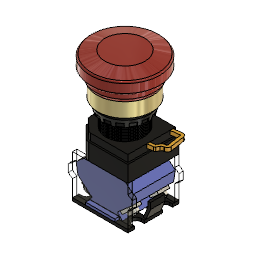
_EStop_LA38 _203 209B.204cfa63-6cc7-4e90-86a4-f45930ce202f (Autodesk Fusion 360 design; units mm, degrees)
Autodesk Fusion 360 part; units mm, degrees
sketch "Sketch1" plane through (0, 0, 0) normal (0, 0, 1) x (1, 0, 0)
  line L0 (16, 14.75) -> (-16, 14.75)
  line L1 (-16, -14.75) -> (16, -14.75)
  line L2 (16, 14.75) -> (-16, -14.75) construction
  line L3 (-16, 14.75) -> (16, -14.75) construction
  line L4 (16, -14.75) -> (16, -11)
  line L5 (16, -5.25) -> (14.375, -5.25)
  arc A0 (14.375, -5.25) -> (14.375, -11) centre (14.375, -8.125) ccw
  line L6 (16, -14.75) -> (16, -11)
  line L7 (16, -11) -> (14.375, -11)
  line L8 (14.25, 3) -> (8.25, 3)
  line L9 (8.25, 3) -> (8.25, -3)
  line L10 (8.25, -3) -> (14.25, -3)
  line L11 (14.25, -3) -> (14.25, 3)
  line L12 (0, -14.75) -> (0, 14.75) construction
  arc A1 (-14.375, -11) -> (-14.375, -5.25) centre (-14.375, -8.125) ccw
  line L13 (-16, -11) -> (-14.375, -11)
  line L14 (-16, -5.25) -> (-14.375, -5.25)
  line L15 (-8.25, -3) -> (-14.25, -3)
  line L16 (-14.25, -3) -> (-14.25, 3)
  line L17 (-14.25, 3) -> (-8.25, 3)
  line L18 (-8.25, 3) -> (-8.25, -3)
  line L19 (-16, 0) -> (16, 0) construction
  arc A2 (-14.375, 5.25) -> (-14.375, 11) centre (-14.375, 8.125) ccw
  line L20 (-16, 5.25) -> (-14.375, 5.25)
  line L21 (-16, 11) -> (-14.375, 11)
  line L22 (16, 11) -> (14.375, 11)
  arc A3 (14.375, 11) -> (14.375, 5.25) centre (14.375, 8.125) ccw
  line L23 (16, 5.25) -> (14.375, 5.25)
  line L24 (-16, 14.75) -> (-16, 11)
  line L25 (-16, 5.25) -> (-16, -5.25)
  line L26 (-16, -11) -> (-16, -14.75)
  line L27 (16, -14.75) -> (16, -11) construction
  line L28 (16, -5.25) -> (16, 5.25)
  line L29 (16, 11) -> (16, 14.75)
  line L30 (16, -5.25) -> (16, 5.25) construction
  line L31 (16, 11) -> (16, 14.75) construction
  dimension "d1" = 32
  dimension "d2" = 29.5
  dimension "d3" = 3.75
  dimension "d4" = 5.75
  dimension "d7" = 6
  dimension "d8" = 6
  constraint horizontal L0
  constraint perpendicular L0 L24
  constraint parallel L0 L1
  constraint parallel L6 L26
  constraint coincident L2 origin
  constraint coincident L3 origin
  constraint perpendicular L1 L4
  constraint perpendicular L5 L28
  constraint tangent L5 A0
  constraint tangent A0 L7
  constraint collinear L6 L28
  constraint horizontal L8
  constraint perpendicular L8 L9
  constraint parallel L8 L10
  constraint parallel L9 L11
  constraint midpoint L1 L12.start
  constraint midpoint L0 L12.end
  constraint symmetric L4.end L12 L13.start
  constraint symmetric L5.start L12 L14.start
  constraint symmetric L5.end L12 A1.end
  constraint symmetric A0 L12 A1
  constraint symmetric A0.end L12 A1.start
  constraint symmetric L8.start L12 L16.end
  constraint symmetric L8.end L12 L17.end
  constraint symmetric L9.end L12 L15.start
  constraint symmetric L10.end L12 L15.end
  constraint symmetric L4.end L19 L22.start
  constraint symmetric L5.start L19 L23.start
  constraint symmetric L5.end L19 A3.end
  constraint symmetric A0 L19 A3
  constraint symmetric A0.end L19 L22.end
  constraint symmetric A1.end L19 A2.start
  constraint symmetric A1.start L19 A2.end
  constraint symmetric A1 L19 A2
  constraint symmetric L13.start L19 L21.start
  constraint symmetric L14.start L19 L20.start
  constraint collinear L24 L25
  constraint collinear L25 L26
  constraint coincident L19.start L25
  constraint collinear L27 L30
  constraint collinear L28 L29
  constraint collinear L30 L31
  constraint coincident L19.end L30
  measures "d1" distance of L1.start L1.end
  measures "d2" distance of L0.end L1.start
  measures "d3" distance of L1.end L4.end
  measures "d4" distance of L4.end L5.start
  measures "d7" distance of L9.end L10.end
  measures "d8" distance of L8.end L9.end
extrude "Extrude1" add sketch "Sketch1" along normal blind 1.75 makes body 1
sketch "Sketch2" plane through (0, -14.75, 0) normal (0, -1, 0) x (1, 0, 0)
  line L0 (-16, 0) -> (16, 0)
  line L1 (16, 0) -> (16, 1.75)
  line L2 (16, 1.75) -> (-16, 1.75)
  line L3 (-16, 1.75) -> (-16, 0)
  line L4 (-16, 1.75) -> (16, 1.75)
  line L5 (16, 24.75) -> (-16, 24.75)
  line L6 (16, 1.75) -> (16, 11.25)
  line L7 (18.5, 13) -> (18.5, 17.5)
  line L8 (18.5, 13) -> (16, 11.25)
  line L9 (18.5, 17.5) -> (16, 19.25)
  line L10 (0, 1.75) -> (0, 24.75) construction
  line L11 (16, 1.75) -> (16, 11.25)
  line L12 (16, 19.25) -> (16, 24.75)
  line L13 (-18.5, 13) -> (-16, 11.25)
  line L14 (-18.5, 13) -> (-18.5, 17.5)
  line L15 (-18.5, 17.5) -> (-16, 19.25)
  line L16 (-16, 24.75) -> (-16, 19.25)
  line L17 (-16, 11.25) -> (-16, 1.75)
  dimension "d11" = 23
  dimension "d12" = 9.5
  dimension "d15" = 4.5
  constraint horizontal L4
  constraint vertical L11
  constraint horizontal L5
  constraint vertical L16
  constraint coincident L2.end L3.start
  constraint coincident L1.end L2.start
  constraint perpendicular L2 L6
  constraint midpoint L2 L10.start
  constraint midpoint L5 L10.end
  constraint perpendicular L5 L10
  constraint collinear L11 L12
  constraint symmetric L6.end L10 L13.end
  constraint symmetric L7.start L10 L13.start
  constraint symmetric L7.end L10 L14.end
  constraint symmetric L9.end L10 L15.end
  constraint collinear L16 L17
  measures "d11" distance of L2.end L5.end
  measures "d12" distance of L1.end L6.end
  measures "d15" distance of L7.start L7.end
extrude "Extrude1'" add sketch "Sketch2" against normal blind 2.5 separate body contours L2 L4 L5 L6 L7 L8 L9 L11 L12 L13 L14 L15 L16 L17 makes body 2 in component "Acryllic Panels"
ref_plane "WorkPlane1" through (0, 0, 0.875) normal (0, 1, 0) x (-1, 0, 0)
mirror "Mirror1" about plane through (0, 0, 0.875) normal (0, 1, 0) of bodies 2 makes body 3 in component "Acryllic Panels"
sketch "Sketch3" plane through (0, -12.25, 0) normal (0, -1, 0) x (1, 0, 0)
  line L0 (-18.5, 13) -> (-16, 11.25)
  line L1 (-16, 11.25) -> (-16, 1.75)
  line L2 (-16, 1.75) -> (16, 1.75)
  line L3 (16, 1.75) -> (16, 11.25)
  line L4 (16, 11.25) -> (18.5, 13)
  line L5 (18.5, 13) -> (18.5, 17.5)
  line L6 (18.5, 17.5) -> (16, 19.25)
  line L7 (16, 19.25) -> (16, 24.75)
  line L8 (16, 24.75) -> (-16, 24.75)
  line L9 (-16, 24.75) -> (-16, 19.25)
  line L10 (-16, 19.25) -> (-18.5, 17.5)
  line L11 (-18.5, 17.5) -> (-18.5, 13)
  line L12 (-16, 0) -> (16, 0)
  line L13 (16, 0) -> (16, 1.75)
  line L14 (16, 1.75) -> (-16, 1.75)
  line L15 (-16, 1.75) -> (-16, 0)
  line L16 (-10.125, 1.75) -> (10.125, 1.75)
  line L17 (0, 1.75) -> (0, 6.5)
  line L18 (-6, 6.5) -> (6, 6.5)
  line L19 (-10.125, 1.75) -> (-6, 6.5)
  line L20 (6, 6.5) -> (10.125, 1.75)
  line L21 (-8.5, 1.75) -> (8.5, 1.75)
  line L22 (-8.5, 1.75) -> (8.5, 1.75)
  line L23 (8.5, 1.75) -> (8.5, 3.25)
  line L24 (8.5, 3.25) -> (-8.5, 3.25)
  line L25 (-8.5, 3.25) -> (-8.5, 1.75)
  line L26 (-6, 6.5) -> (-6, 12) construction
  line L27 (-18.5, 14) -> (-15.5, 14) construction
  line L28 (-15.5, 12) -> (-7.3614, 4.9323)
  line L29 (-15.5, 12) -> (-16.5, 18.25)
  line L30 (-9, 24.75) -> (-16.5, 18.25)
  line L31 (15.5, 12) -> (7.3614, 4.9323)
  line L32 (15.5, 12) -> (16.5, 18.25)
  line L33 (9, 24.75) -> (16.5, 18.25)
  line L34 (-9, 24.75) -> (9, 24.75)
  line L35 (-16, 11.25) -> (-18.5, 13)
  line L36 (-18.5, 13) -> (-18.5, 17.5)
  line L37 (-18.5, 17.5) -> (-16, 19.25)
  line L38 (-16, 19.25) -> (-16, 24.75)
  line L39 (-16, 24.75) -> (16, 24.75)
  line L40 (16, 24.75) -> (16, 19.25)
  line L41 (16, 19.25) -> (18.5, 17.5)
  line L42 (18.5, 17.5) -> (18.5, 13)
  line L43 (18.5, 13) -> (16, 11.25)
  line L44 (16, 11.25) -> (16, 1.75)
  line L45 (16, 1.75) -> (-16, 1.75)
  line L46 (-16, 1.75) -> (-16, 11.25)
  point P0 (0, 1.75)
  point P1 (0, 1.75)
  dimension "d20" = 20.25
  dimension "d21" = 4.75
  dimension "d22" = 12
  dimension "d23" = 17
  dimension "d24" = 1.5
  dimension "d25" = 5.5
  dimension "d26" = 3
  constraint midpoint L16 P1
  constraint coincident L14 P1
  constraint parallel L2 L16
  constraint coincident P1 P0
  constraint perpendicular L2 L17
  constraint midpoint L17.end L18
  constraint perpendicular L17 L18
  constraint midpoint L21 P1
  constraint perpendicular L17 L21
  constraint horizontal L22
  constraint vertical L23
  constraint horizontal L24
  constraint vertical L25
  constraint perpendicular L18 L26
  constraint coincident L11 L27.start
  constraint perpendicular L11 L27
  constraint coincident L19 L28.end
  constraint perpendicular L19 L28
  constraint coincident L8 L30.start
  constraint symmetric L17 L28.start L31.start
  constraint symmetric L17 L28.end L31.end
  constraint symmetric L17 L29.end L32.end
  constraint symmetric L17 L30.start L33.start
  measures "d20" distance of L16.start L16.end
  measures "d21" distance of P1 L17.end
  measures "d22" distance of L18.start L18.end
  measures "d23" distance of L21.start L21.end
  measures "d24" distance of L21.start L24.end
  measures "d25" distance of L18.start L26.end
  measures "d26" distance of L27.start L27.end
extrude "Extrude2" cut sketch "Sketch3" along normal blind 2.5 contours L2 L14 L16 L17 L21 L22 L24 L25 L45 | L2 L14 L16 L17 L21 L22 L23 L24 L45 bodies 2 in component "Acryllic Panels"
extrude "Extrude1''" add sketch "Sketch3" along normal blind 2.5 separate body contours L2 L14 L16 L17 L21 L22 L24 L25 L45 | L2 L14 L16 L17 L21 L22 L23 L24 L45 makes body 4 in component "Inner Mechanism Block"
extrude "Extrude2'" add sketch "Sketch3" against normal blind 12.25 contours L2 L14 L16 L17 L18 L19 L24 L25 L45 | L2 L14 L16 L17 L21 L22 L24 L25 L45 | L8 L18 L19 L20 L28 L29 L30 L31 L32 L33 L34 L39 | L2 L14 L16 L17 L21 L22 L23 L24 L45 | L2 L14 L16 L17 L18 L20 L23 L24 L45 bodies 4 in component "Inner Mechanism Block"
mirror "Mirror1'" about plane through (0, 0, 0.875) normal (0, 1, 0) of bodies 4 merged in component "Inner Mechanism Block"
copy_body "Body->Comp1" bodies 1 removing the originals makes body 5 in component "Bottom Base"
sketch "Sketch4" plane through (0, 0, 0) normal (0, 1, 0) x (1, 0, 0)
  line L0 (-8.25, 0) -> (-8.25, -1.75)
  line L1 (-8.25, -1.75) -> (8.25, -1.75)
  line L2 (8.25, -1.75) -> (8.25, 0)
  line L3 (8.25, 0) -> (-8.25, 0)
  line L4 (16, -1.75) -> (16, 0)
  line L5 (16, 0) -> (14.25, 0)
  line L6 (14.25, 0) -> (14.25, -1.75)
  line L7 (14.25, -1.75) -> (16, -1.75)
  line L8 (-16, 0) -> (-16, -1.75)
  line L9 (-16, -1.75) -> (-14.25, -1.75)
  line L10 (-14.25, -1.75) -> (-14.25, 0)
  line L11 (-14.25, 0) -> (-16, 0)
  line L12 (-16, -1.75) -> (-16, -7.75)
  line L13 (-16, -7.75) -> (-18.5, -7.75)
  line L14 (-16, -1.75) -> (-18.5, -7.75)
  line L15 (-18.5, -7.75) -> (-18.5, -11.25)
  line L16 (-17, -8.05) -> (-17, -11.25)
  line L17 (-18.5, -11.25) -> (-17, -11.25)
  line L18 (-14.25, -1.75) -> (-17, -8.05)
  line L19 (0, -1.75) -> (0, -4) construction
  line L20 (14.25, -1.75) -> (17, -8.05)
  line L21 (16, -1.75) -> (18.5, -7.75)
  line L22 (17, -8.05) -> (17, -11.25)
  line L23 (18.5, -7.75) -> (18.5, -11.25)
  line L24 (18.5, -11.25) -> (17, -11.25)
  dimension "d37" = 6
  dimension "d38" = 2.5
  dimension "d39" = 3.5
  dimension "d40" = -1.5
  constraint coincident L8.end L9.start
  constraint perpendicular L9 L12
  constraint perpendicular L12 L13
  constraint perpendicular L13 L15
  constraint perpendicular L16 L17
  constraint coincident L9.end L10.start
  constraint midpoint L1 L19.start
  constraint perpendicular L1 L19
  constraint symmetric L13.end L19 L21.end
  constraint symmetric L8.end L19 L4.start
  constraint symmetric L15.end L19 L23.end
  constraint symmetric L16.start L19 L20.end
  constraint symmetric L16.end L19 L22.end
  constraint symmetric L9.end L19 L6.end
  measures "d37" distance of L8.end L12.end
  measures "d38" distance of L12.end L13.end
  measures "d39" distance of L13.end L15.end
extrude "Extrude1'''" add sketch "Sketch4" along normal mid plane 8.4 contours L7 L20 L21 L22 L23 L24 | L9 L12 L18 | L12 L13 L14 L18 | L13 L15 L16 L17 L18 bodies 5 in component "Bottom Base"
sketch "Sketch5" plane through (0, -14.75, 0) normal (0, -1, 0) x (1, 0, 0)
  line L0 (8.5, 3.25) -> (8.5, 1.75)
  line L1 (8.5, 1.75) -> (16, 1.75)
  line L2 (16, 1.75) -> (16, 11.25)
  line L3 (16, 11.25) -> (18.5, 13)
  line L4 (18.5, 13) -> (18.5, 17.5)
  line L5 (18.5, 17.5) -> (16, 19.25)
  line L6 (16, 19.25) -> (16, 24.75)
  line L7 (16, 24.75) -> (-16, 24.75)
  line L8 (-16, 24.75) -> (-16, 19.25)
  line L9 (-16, 19.25) -> (-18.5, 17.5)
  line L10 (-18.5, 17.5) -> (-18.5, 13)
  line L11 (-18.5, 13) -> (-16, 11.25)
  line L12 (-16, 11.25) -> (-16, 1.75)
  line L13 (-16, 1.75) -> (-8.5, 1.75)
  line L14 (-8.5, 1.75) -> (-8.5, 3.25)
  line L15 (-8.5, 3.25) -> (8.5, 3.25)
  line L16 (-16, 1.75) -> (16, 1.75)
  line L17 (-16, 0) -> (16, 0)
  line L18 (16, 0) -> (16, 1.75)
  line L19 (16, 1.75) -> (-16, 1.75)
  line L20 (-16, 1.75) -> (-16, 0)
extrude "Extrude3" cut sketch "Sketch5" against normal blind 29.5 contours L0 L14 L15 L16 L19 bodies 3 in component "Acryllic Panels"
ref_plane "WorkPlane2" through (14.2174, 0, 5.2573) normal (0.655687, 0, -0.755033) x (-0.755033, 0, -0.655687)
sketch "Sketch6" plane through (3.5097, 0, -4.0415) normal (0.655687, 0, -0.755033) x (-0.755033, 0, -0.655687)
  line L0 (-19.5713, -12.25) -> (-8.7922, -12.25)
  line L1 (-8.7922, -12.25) -> (-8.7922, 12.25)
  line L2 (-8.7922, 12.25) -> (-19.5713, 12.25)
  line L3 (-19.5713, 12.25) -> (-19.5713, -12.25)
  ellipse E0 centre (-10.8536, -8.125) end of major axis (-10.8536, -5.25) minor radius 2.1707 (-10.8536, -11) -> (-10.8536, -5.25) ccw
  line L4 (-10.8536, -8.125) -> (-8.7922, -8.125)
  line L5 (-8.7922, -8.125) -> (-13.0422, -8.125)
  circle A0 centre (-13.0422, -8.125) radius 2.75
  line L6 (-8.7922, 0) -> (-10.2486, 0) construction
  circle A1 centre (-13.0422, 8.125) radius 2.75
  dimension "d46" = 4.25
  dimension "d47" = 5.5
  constraint coincident E0.centre L4.start
  constraint coincident L1 L4.end
  constraint perpendicular L1 L4
  constraint perpendicular L1 L5
  constraint coincident L5.end A0.centre
  constraint midpoint L1 L6.start
  constraint perpendicular L1 L6
  constraint symmetric A0 L6 A1
  measures "d46" distance of L4.end L5.end
  measures "d47" diameter of A0
extrude "Extrude1''''" add sketch "Sketch6" against normal blind 4.25 separate body contours A0 | A1 makes body 6 at (10.3621, 7.8512, 3.7855) makes body 7 at (9.4254, -8.2621, 4.8484) in component "Screw Terminals"
ref_plane "WorkPlane3" through (11.7178, 8.125, 6.3977) normal (0.655687, 0, -0.755033) x (-0.755033, 0, -0.655687)
sketch "Sketch7" plane through (1.8705, 0, -2.1539) normal (0.655687, 0, -0.755033) x (-0.755033, 0, -0.655687)
  circle A0 centre (-13.0422, 8.125) radius 2.75
  circle A1 centre (-13.0422, -8.125) radius 2.75
  line L0 (-16.2922, -4.875) -> (-9.7922, -4.875)
  line L1 (-9.7922, -4.875) -> (-9.7922, -11.375)
  line L2 (-9.7922, -11.375) -> (-16.2922, -11.375)
  line L3 (-16.2922, -11.375) -> (-16.2922, -4.875)
  line L4 (-16.2922, -4.875) -> (-9.7922, -11.375) construction
  line L5 (-9.7922, -4.875) -> (-16.2922, -11.375) construction
  line L6 (-16.2922, 11.375) -> (-9.7922, 11.375)
  line L7 (-9.7922, 11.375) -> (-9.7922, 4.875)
  line L8 (-9.7922, 4.875) -> (-16.2922, 4.875)
  line L9 (-16.2922, 4.875) -> (-16.2922, 11.375)
  line L10 (-16.2922, 11.375) -> (-9.7922, 4.875) construction
  line L11 (-9.7922, 11.375) -> (-16.2922, 4.875) construction
  point P0 (-13.0422, -8.125)
  point P1 (-13.0422, 8.125)
  dimension "d51" = 6.5
  dimension "d52" = 6.5
  dimension "d53" = 6.5
  dimension "d54" = 6.5
  constraint horizontal L0
  constraint perpendicular L0 L1
  constraint parallel L0 L2
  constraint parallel L1 L3
  constraint coincident L4 P0
  constraint coincident L5 P0
  constraint coincident P0 A1.centre
  constraint horizontal L6
  constraint perpendicular L6 L7
  constraint parallel L6 L8
  constraint parallel L7 L9
  constraint coincident L10 P1
  constraint coincident L11 P1
  constraint coincident A0.centre P1
  measures "d51" distance of L1.end L2.end
  measures "d52" distance of L0.end L1.end
  measures "d53" distance of L7.end L8.end
  measures "d54" distance of L6.end L7.end
extrude "Extrude2''" cut sketch "Sketch7" against normal blind 1.75 contours A0 | A1 bodies 6 7 in component "Screw Terminals"
extrude "Extrude3'" add sketch "Sketch7" against normal blind 1.75 contours A0 | A1 | L0 L1 L2 L3 | L6 L7 L8 L9 bodies 6 7 in component "Screw Terminals"
sketch "Sketch8" plane through (3.5097, 0, -4.0415) normal (0.655687, 0, -0.755033) x (0, 1, 0)
  circle A0 centre (-8.125, 13.0422) radius 2.75
  circle A1 centre (8.125, 13.0422) radius 2.75
  line L0 (-8.75, 16) -> (-7.5565, 10.3516) construction
  line L1 (-5.404, 13.4408) -> (-10.846, 12.6435) construction
  line L2 (-8.125, 13.0422) -> (8.125, 13.0422)
  line L3 (0, 13.0422) -> (0, 14.5)
  line L4 (7.5, 10.0843) -> (7.5, 16)
  line L5 (8.75, 16) -> (8.75, 10.0843)
  line L6 (7.5, 16) -> (8.75, 16)
  line L7 (8.75, 10.0843) -> (7.5, 10.0843)
  line L8 (11.25, 12.5843) -> (5, 12.5843)
  line L9 (5, 13.5) -> (11.25, 13.5)
  line L10 (5, 12.5843) -> (5, 13.5)
  line L11 (-8.75, 15.7202) -> (-8.75, 13.5)
  line L12 (-8.75, 12.5843) -> (-8.75, 10.3641)
  line L13 (-5.4134, 13.5) -> (-7.5, 13.5)
  line L14 (-8.75, 13.5) -> (-10.8366, 13.5)
  line L15 (-7.5, 16) -> (-8.125, 13.0422) construction
  line L16 (-8.2217, 12.5843) -> (-8.6935, 10.3516) construction
  line L17 (-10.8366, 12.5843) -> (-8.75, 12.5843)
  line L18 (-7.5, 12.5843) -> (-5.4134, 12.5843)
  line L19 (-10.846, 13.4408) -> (-7.5, 12.9506) construction
  line L20 (-5.404, 12.6435) -> (-5, 12.5843) construction
  line L21 (-7.5, 10.3641) -> (-7.5, 12.5843)
  line L22 (-7.5, 12.9506) -> (-7.5, 15.7202)
  point P0 (-8.125, 13.0422)
  point P1 (-8.125, 13.0422)
  constraint parallel L11 L22
  constraint coincident P1 L15
  constraint coincident L0 P1
  constraint coincident P0 A0.centre
  constraint horizontal L13
  constraint parallel L13 L18
  constraint coincident L1 P1
  constraint coincident P1 L19
  constraint coincident P1 P0
  constraint coincident A1.centre L2.end
  constraint midpoint L2 L3.start
  constraint perpendicular L2 L3
  constraint symmetric L15.start L3 L4.end
  constraint symmetric L0.start L3 L5.start
  constraint symmetric L20.end L3 L8.end
  constraint coincident A0 L11.start
  constraint coincident A0 L22.end
  constraint coincident L13.end L22
  constraint collinear L15 L16
  constraint collinear L17 L18
  constraint coincident A0 L19.start
  constraint coincident A0 L14.end
  constraint coincident A0 L17.start
  constraint coincident A0 L1.end
  constraint coincident A0 L16.end
  constraint coincident A0 L0.end
  constraint coincident A0 L21.start
  constraint coincident A0 L12.end
  constraint coincident A0 L18.end
  constraint coincident A0 L1.start
  constraint coincident A0 L13.start
  constraint coincident A0 L20.start
  constraint collinear L19 L20
  constraint collinear L21 L22
extrude "Extrude4" cut sketch "Sketch8" against normal blind 0.75 contours A0 L2 L13 L22 | A0 L2 L11 L12 L14 L17 L18 L21 L22 | A1 L5 L8 L9 | A1 L4 L5 L9 | L4 L5 L8 L9 | A1 L4 L5 L8 | A1 L2 L4 L9 | A1 L2 L4 L8 bodies 6 7 in component "Screw Terminals"
chamfer "Chamfer1" distance 0.75 angle 45 8 edges at (14.779, -10.1289, 5.7449) (14.779, -6.1211, 5.7449) (11.935, -6.1211, 3.2752) (11.935, -10.1289, 3.2752) (14.779, 6.1211, 5.7449) (11.935, 6.1211, 3.2752) (11.935, 10.1289, 3.2752) (14.779, 10.1289, 5.7449) on bodies 6 7 in component "Screw Terminals"
ref_plane "WorkPlane4" through (0, 0, 0.875) normal (1, 0, 0) x (0, 1, 0)
mirror "Mirror1''" about plane through (0, 0, 0.875) normal (1, 0, 0) of bodies 6 7 makes body 8 at (-11.3883, 9.2083, 8.4293) makes body 9 at (-11.3883, -7.0417, 8.4293) in component "Screw Terminals"
sketch "Sketch9" plane through (0, 0, 24.75) normal (0, 0, 1) x (-1, 0, 0)
  line L0 (9, 12.25) -> (-9, 12.25)
  line L1 (-9, 12.25) -> (-9, -12.25)
  line L2 (-9, -12.25) -> (9, -12.25)
  line L3 (9, -12.25) -> (9, 12.25)
  line L4 (-16, -14.75) -> (16, -14.75)
  line L5 (16, -14.75) -> (16, -12.25)
  line L6 (16, -12.25) -> (-16, -12.25)
  line L7 (-16, -12.25) -> (-16, -14.75)
  line L8 (16, 14.75) -> (-16, 14.75)
  line L9 (-16, 14.75) -> (-16, 12.25)
  line L10 (-16, 12.25) -> (16, 12.25)
  line L11 (16, 12.25) -> (16, 14.75)
  line L12 (16, -12.25) -> (16, 12.25)
  line L13 (16, 7) -> (16, -7)
  line L14 (16, 0) -> (-9, 0) construction
  line L15 (-16, 12.25) -> (8, 12.25)
  line L16 (16, -7) -> (16, 7)
  line L17 (-16, 12.25) -> (8, 12.25)
  line L18 (-16, 12.25) -> (-16, -12.25)
  line L19 (-16, -14.75) -> (6.5827, -14.75)
  line L20 (-16, 14.75) -> (6.5827, 14.75)
  line L21 (9.018, 13.7638) -> (16, 7)
  line L22 (16, -7) -> (9.018, -13.7638)
  arc A0 (9.018, 13.7638) -> (6.5827, 14.75) centre (6.5827, 11.25) ccw
  arc A1 (6.5827, -14.75) -> (9.018, -13.7638) centre (6.5827, -11.25) ccw
  point P0 (16, 0)
  point P1 (8, -14.75)
  point P2 (8, 14.75)
  dimension "d65" = 14
  dimension "d66" = 24
  dimension "d67" = 24
  dimension "d68" = 3.5
  constraint coincident L6.end L7.start
  constraint coincident L5.end L6.start
  constraint coincident L10.end L11.start
  constraint midpoint L13 P0
  constraint coincident L12 P0
  constraint parallel L12 L13
  constraint coincident P0 L14.start
  constraint midpoint L1 L14.end
  constraint perpendicular L1 L14
  constraint symmetric L6.end L14 L9.end
  constraint symmetric L13.start L14 L13.end
  constraint symmetric L13.end L14 L13.start
  constraint coincident L9.end L10.start
  constraint coincident L4.start L7.end
  constraint perpendicular L7 L19
  constraint coincident L8.end L9.start
  constraint perpendicular L9 L20
  constraint coincident P2 L20
  constraint coincident P2 L21
  constraint tangent L20 A0
  constraint tangent L21 A0
  constraint coincident P1 L22
  constraint coincident P1 L19
  constraint tangent L22 A1
  constraint tangent L19 A1
  constraint equal A0 A1
  measures "d65" distance of L13.start L13.end
  measures "d66" distance of L4.start P1
  measures "d67" distance of L8.end P2
  measures "d68" radius of A0
extrude "Extrude1'''''" add sketch "Sketch9" along normal blind 9.5 separate body contours L0 L1 L2 L3 L6 L10 L15 L17 | L3 L6 L10 L12 L13 L16 L21 L22 | L0 L8 L9 L10 L15 L17 L20 L21 A0 | L2 L4 L6 L7 L19 L22 A1 | L1 L6 L10 L15 L17 L18 makes body 10 in component "Main Block"
sketch "Sketch10" plane through (0, 0, 34.25) normal (0, 0, 1) x (-1, 0, 0)
  line L0 (-16, 14.75) -> (-16, -14.75)
  line L1 (-16, -14.75) -> (6.5827, -14.75)
  arc A0 (6.5827, -14.75) -> (9.018, -13.7638) centre (6.5827, -11.25) ccw
  line L2 (9.018, -13.7638) -> (16, -7)
  line L3 (16, -7) -> (16, 7)
  line L4 (16, 7) -> (9.018, 13.7638)
  arc A1 (9.018, 13.7638) -> (6.5827, 14.75) centre (6.5827, 11.25) ccw
  line L5 (6.5827, 14.75) -> (-16, 14.75)
  line L6 (6.5827, 13.75) -> (-15, 13.75)
  line L7 (-15, 13.75) -> (-15, -13.75)
  line L8 (-15, -13.75) -> (6.5827, -13.75)
  arc A2 (6.5827, -13.75) -> (8.3222, -13.0456) centre (6.5827, -11.25) ccw
  line L9 (8.3222, -13.0456) -> (15, -6.5765)
  line L10 (15, -6.5765) -> (15, 6.5765)
  line L11 (15, 6.5765) -> (8.3222, 13.0456)
  arc A3 (8.3222, 13.0456) -> (6.5827, 13.75) centre (6.5827, 11.25) ccw
  dimension "d71" = -1
extrude "Extrude2'''" add sketch "Sketch10" along normal blind 4 contours L6 L7 L8 A2 L9 L10 L11 A3 bodies 10 in component "Main Block"
extrude "Extrude3''" cut 1 faces at (-2.4538, -12.25, 18.1441) along direction (0, 1, 0) blind 0.1 on bodies 4 bodies 4 in component "Inner Mechanism Block"
extrude "Extrude4'" cut 1 faces at (-2.4538, 12.25, 18.1441) along direction (0, -1, 0) blind 0.1 on bodies 4 bodies 4 in component "Inner Mechanism Block"
sketch "Sketch11" plane through (0, 0, 38.25) normal (0, 0, 1) x (-1, 0, 0)
  arc A0 (8.3222, 13.0456) -> (6.5827, 13.75) centre (6.5827, 11.25) ccw
  line L0 (6.5827, 13.75) -> (-15, 13.75)
  line L1 (-15, 13.75) -> (-15, -13.75)
  line L2 (-15, -13.75) -> (6.5827, -13.75)
  arc A1 (6.5827, -13.75) -> (8.3222, -13.0456) centre (6.5827, -11.25) ccw
  line L3 (8.3222, -13.0456) -> (15, -6.5765)
  line L4 (15, -6.5765) -> (15, 6.5765)
  line L5 (15, 6.5765) -> (8.3222, 13.0456)
  line L6 (15, 0) -> (1, 0)
  circle A2 centre (1, 0) radius 10.75
  dimension "d78" = 14
  dimension "d79" = 21.5
  constraint midpoint L4 L6.start
  constraint perpendicular L4 L6
  constraint coincident L6.end A2.centre
  measures "d78" distance of L6.start L6.end
  measures "d79" diameter of A2
extrude "Extrude1''''''" add sketch "Sketch11" along normal blind 8.5 separate body contours A2 makes body 11 in component "Button Threaded Base"
sketch "Sketch12" plane through (0, 0, 46.75) normal (0, 0, 1) x (-1, 0, 0)
  circle A0 centre (1, 0) radius 10.75
  circle A1 centre (1, 0) radius 13
  dimension "d82" = 26
  constraint concentric A0 A1
  measures "d82" diameter of A1
ref_plane "WorkPlane5" through (-1, 0, 51.25) normal (0, 0, 1) x (-1, 0, 0)
sketch "Sketch13" plane through (0, 0, 51.25) normal (0, 0, 1) x (1, 0, 0)
  circle A0 centre (-1, 0) radius 14.125
  dimension "d84" = 28.25
  measures "d84" diameter of A0
loft "Loft1" add profiles "Sketch12", "Sketch13" section 1 contours A0 | A1 section 2 bodies 11 in component "Button Threaded Base"
extrude "Extrude2''''" add 1 faces at (0.1003, -3.8885, 51.25) along direction (0, 0, 1) blind 2 on bodies 11 bodies 11 in component "Button Threaded Base"
sketch "Sketch14" plane through (0, 13.75, 0) normal (0, 1, 0) x (-1, 0, 0)
  line L0 (-15, 34.25) -> (6.5827, 34.25)
  line L1 (6.5827, 34.25) -> (6.5827, 38.25)
  line L2 (6.5827, 38.25) -> (-15, 38.25)
  line L3 (-15, 38.25) -> (-15, 34.25)
  line L4 (14, 46.75) -> (-12, 46.75)
  line L5 (-13.125, 51.25) -> (15.125, 51.25)
  line L6 (-12, 46.75) -> (14, 46.75)
  line L7 (1, 46.75) -> (1, 49.25)
  line L8 (2.75, 49.25) -> (-0.75, 49.25)
  line L9 (-0.75, 49.25) -> (-0.75, 46.75)
  line L10 (-0.75, 46.75) -> (2.75, 46.75)
  line L11 (2.75, 46.75) -> (2.75, 49.25)
  line L12 (2.75, 49.25) -> (-0.75, 46.75) construction
  line L13 (-0.75, 49.25) -> (2.75, 46.75) construction
  point P0 (1, 48)
  dimension "d87" = 2.5
  dimension "d88" = 3.5
  constraint coincident L4.end L6.start
  constraint coincident L4.start L6.end
  constraint midpoint L4 L7.start
  constraint perpendicular L6 L7
  constraint horizontal L8
  constraint perpendicular L8 L9
  constraint parallel L8 L10
  constraint parallel L9 L11
  constraint coincident L12 P0
  constraint coincident L13 P0
  constraint midpoint L7 P0
  measures "d87" distance of L7.start L7.end
  measures "d88" distance of L9.end L10.end
extrude "Extrude3'''" cut sketch "Sketch14" against normal blind 1.25 contours L4 L6 L7 L8 L10 L11 | L4 L6 L7 L8 L9 L10 bodies 11 in component "Button Threaded Base"
pattern_circular "C-Pattern1" count 15 over 360 about axis through (-1, 0, 51.25) along (0, 0, -1) of "Extrude3'''" in component "Button Threaded Base"
sketch "Sketch15" plane through (0, 0, 53.25) normal (0, 0, 1) x (-1, 0, 0)
  circle A0 centre (1, 0) radius 14.125
  circle A1 centre (1, 0) radius 15.625
  dimension "d93" = 31.25
  constraint concentric A0 A1
  measures "d93" diameter of A1
extrude "Extrude1'''''''" add sketch "Sketch15" along normal blind 8.75 separate body contours A0 | A1 makes body 12 in component "Gold Band"
thread "Thread1" "ISO Metric profile 22.0 M22x0.75 M22x0.75 6g" major diameter 21.908 minor diameter 21.0445 pitch 0.75 angle 60 modelled right hand crest width 0.1036 on face at (-11.7366, 0.5358, 43.9167) crest through (-11.954, 0, 38.0625) on bodies 11 in component "Button Threaded Base"
sketch "Sketch16" plane through (0, 0, 0) normal (0, 1, 0) x (1, 0, 0)
  line L0 (14.625, -62) -> (14.625, -53.25)
  line L1 (14.625, -53.25) -> (-16.625, -53.25)
  line L2 (-16.625, -53.25) -> (-16.625, -62)
  line L3 (-16.625, -62) -> (14.625, -62)
  line L4 (-1, -62) -> (15.25, -62)
  line L5 (15.25, -62) -> (15.25, -63.75)
  line L6 (-1, -63.75) -> (16, -63.75)
  line L7 (15.25, -62) -> (16, -63.75)
  line L8 (17.5, -67.75) -> (19, -67.75)
  line L9 (16, -63.75) -> (16, -66.25)
  arc A0 (16, -66.25) -> (17.5, -67.75) centre (17.5, -66.25) ccw
  line L10 (19, -67.75) -> (19, -74.5)
  line L11 (-1, -74.5) -> (-1, -76.5)
  line L12 (-1, -76.5) -> (10.5, -76.5)
  line L13 (10.5, -76.5) -> (19, -74.5)
  line L14 (-1, -62) -> (-1, -74.5)
  point P0 (16, -67.75)
  dimension "d98" = 16.25
  dimension "d99" = 1.75
  dimension "d100" = 17
  dimension "d103" = 3
  dimension "d104" = 1.5
  dimension "d105" = 6.75
  dimension "d106" = 11.5
  constraint midpoint L3 L4.start
  constraint perpendicular L0 L4
  constraint perpendicular L4 L5
  constraint perpendicular L5 L6
  constraint perpendicular L8 L9
  constraint coincident P0 L9
  constraint coincident P0 L8
  constraint tangent L9 A0
  constraint tangent L8 A0
  constraint perpendicular L8 L10
  constraint perpendicular L6 L11
  constraint perpendicular L10 L12
  constraint perpendicular L3 L14
  measures "d98" distance of L4.start L4.end
  measures "d99" distance of L4.end L5.end
  measures "d100" distance of L6.start L6.end
  measures "d103" distance of P0 L8.end
  measures "d104" radius of A0
  measures "d105" distance of L8.end L10.end
  measures "d106" distance of L11.end L12.end
revolve "Revolve1" add sketch "Sketch16" angle 360 about axis through (-1, 0, 62) along (0, 0, 1) separate body contours L3 L4 L5 L6 L14 | L5 L6 L7 | L6 L8 L9 A0 L10 L11 L12 L13 L14 makes body 13 in component "Red Cap"
fillet "Fillet1" radius 1 2 edges at (-19.6465, -7.2323, 74.5) (-19.6465, -7.2323, 67.75) on bodies 13 in component "Red Cap"
sketch "Sketch17" plane through (0, 0, 38.25) normal (0, 0, 1) x (-1, 0, 0)
  arc A0 (8.3222, 13.0456) -> (6.5827, 13.75) centre (6.5827, 11.25) ccw
  line L0 (6.5827, 13.75) -> (-15, 13.75)
  line L1 (-15, 13.75) -> (-15, -13.75)
  line L2 (-15, -13.75) -> (6.5827, -13.75)
  arc A1 (6.5827, -13.75) -> (8.3222, -13.0456) centre (6.5827, -11.25) ccw
  line L3 (8.3222, -13.0456) -> (15, -6.5765)
  line L4 (15, -6.5765) -> (15, 6.5765)
  line L5 (15, 6.5765) -> (8.3222, 13.0456)
  line L6 (-15, -13.75) -> (-15, -12.25)
  line L7 (-15, -12.25) -> (-15, -13.25)
  line L8 (-15, -12.25) -> (-19.9488, -12.9635)
  line L9 (-22.2138, -11.2693) -> (-23.4267, -2.8563)
  line L10 (-21.7325, -0.5914) -> (-21.4851, -0.5557)
  line L11 (-18.4932, 2.4015) -> (-15, 2.9051)
  arc A2 (-22.2138, -11.2693) -> (-19.9488, -12.9635) centre (-20.2342, -10.9839) ccw
  arc A3 (-21.7325, -0.5914) -> (-23.4267, -2.8563) centre (-21.4471, -2.5709) ccw
  line L12 (-21.4851, -0.5557) -> (-21.5796, -0.5693)
  line L13 (-20.1573, 0.3691) -> (-19.2044, 1.9322)
  arc A4 (-21.5796, -0.5693) -> (-20.1573, 0.3691) centre (-21.865, 1.4102) ccw
  arc A5 (-18.4932, 2.4015) -> (-19.2044, 1.9322) centre (-18.3506, 1.4117) ccw
  line L14 (-15.2497, -10.5179) -> (-20.1985, -11.2314)
  arc A6 (-20.4817, -11.0196) -> (-20.1985, -11.2314) centre (-20.2342, -10.9839) ccw
  line L15 (-20.4817, -11.0196) -> (-21.6946, -2.6066)
  arc A7 (-21.4828, -2.3235) -> (-21.6946, -2.6066) centre (-21.4471, -2.5709) ccw
  line L16 (-21.4828, -2.3235) -> (-21.3299, -2.3014)
  line L17 (-21.3299, -2.3014) -> (-21.2354, -2.2878)
  arc A8 (-21.2354, -2.2878) -> (-21.0339, -2.2465) centre (-21.4851, -0.5557) ccw
  arc A9 (-21.0339, -2.2465) -> (-18.6631, -0.5418) centre (-21.865, 1.4102) ccw
  line L18 (-18.6631, -0.5418) -> (-17.894, 0.7198)
  line L19 (-17.894, 0.7198) -> (-14.7503, 1.173)
  line L20 (-16.0348, -10.6311) -> (-15, -10.4819)
  point P0 (-21.9284, -13.2489)
  point P1 (-23.712, -0.8768)
  dimension "d110" = 1.5
  dimension "d111" = 1
  dimension "d112" = 7
  dimension "d113" = 12.5
  dimension "d116" = 2
  dimension "d117" = 2
  dimension "d118" = 2
  dimension "d119" = 1
  dimension "d120" = 1.75
  constraint coincident L1.end L2.start
  constraint perpendicular L2 L6
  constraint parallel L1 L7
  constraint perpendicular L8 L9
  constraint perpendicular L9 L10
  constraint coincident P0 L8
  constraint coincident P0 L9
  constraint tangent L8 A2
  constraint tangent L9 A2
  constraint coincident P1 L9
  constraint coincident P1 L10
  constraint tangent L9 A3
  constraint tangent L10 A3
  constraint parallel L10 L12
  constraint tangent L13 A4
  constraint tangent L12 A4
  constraint tangent L11 A5
  constraint tangent L13 A5
  constraint coincident L1 L11.end
  constraint coincident L14 L20.start
  constraint parallel L14 L20
  constraint coincident L1 L20.end
  measures "d110" distance of L1.end L6.end
  measures "d111" distance of L6.end L7.end
  measures "d112" distance of L6.end P0
  measures "d113" distance of P0 P1
  measures "d116" radius of A2
  measures "d117" radius of A3
  measures "d118" radius of A4
  measures "d119" radius of A5
extrude "Extrude1''''''''" add sketch "Sketch17" against normal blind 2.25 separate body contours L1 L8 L9 L10 L11 A2 A3 L13 A4 A5 L14 A6 L15 A7 L16 L17 A8 A9 L18 L19 L20 makes body 14 in component "Set Latch"
component "Button" placed x (1, 0, 0) y (0, 1, 0) z (0, 0, 1) at (0, 0, 0)
component "Base" placed x (1, 0, 0) y (0, 1, 0) z (0, 0, 1) at (0, 0, 0)
component "Button Threaded Base" placed x (1, 0, 0) y (0, 1, 0) z (0, 0, 1) at (0.9935, -0.4251, 0) in component "Button"
component "Gold Band" placed x (1, 0, 0) y (0, 1, 0) z (0, 0, 1) at (0.9935, -0.4251, 0) in component "Button"
component "Red Cap" placed x (1, 0, 0) y (0, 1, 0) z (0, 0, 1) at (0.9935, -0.4251, 0) in component "Button"
component "Bottom Base" placed x (1, 0, 0) y (0, 1, 0) z (0, 0, 1) at (0, 0, 0) in component "Base"
component "Inner Mechanism Block" placed x (1, 0, 0) y (0, 1, 0) z (0, 0, 1) at (0, 0, 0) in component "Base"
component "Acryllic Panels" placed x (1, 0, 0) y (0, 1, 0) z (0, 0, 1) at (0, 0, 0) in component "Base"
component "Screw Terminals" placed x (1, 0, 0) y (0, 1, 0) z (0, 0, 1) at (0, 0, 0) in component "Base"
component "Main Block" placed x (1, 0, 0) y (0, 1, 0) z (0, 0, 1) at (0, 0, 0) in component "Base"
component "Set Latch" placed x (1, 0, 0) y (0, 1, 0) z (0, 0, 1) at (0, 0, 0) in component "Base"
equation "d98 = ( 32.5 / 2 ) * 1 mm"
equation "d100 = ( 34 / 2 ) * 1 mm"
equation "d106 = ( 23 / 2 ) * 1 mm"
